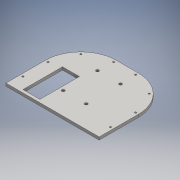
# Autodesk Inventor part: back_platform
Saved by Autodesk Inventor 2016 (Build 200138000, 138)
## iProperties
Created: 2015-09-09
Part Number: back_platform
Material: Generic
Document SubType Name: Modeling
Designer: oscar
Density: 1 g/cm^3
Appearance: Default
Author: oscar
Autodesk Inventor part; units mm, degrees
ref_plane "YZ Plane" through (0, 0, 0) normal (1, 0, 0) x (0, 1, 0)
ref_plane "XZ Plane" through (0, 0, 0) normal (0, 1, 0) x (-1, 0, 0)
ref_plane "XY Plane" through (0, 0, 0) normal (0, 0, 1) x (1, 0, 0)
sketch "Sketch1" plane through (0, 0, 0) normal (0, 0, 1) x (1, 0, 0)
  arc A0 (2041.1632, 1770.0189) -> (1915.1632, 1644.0189) centre (2041.1632, 1644.0189) ccw
  arc A1 (2245.1632, 1644.0189) -> (2119.1632, 1770.0189) centre (2119.1632, 1644.0189) ccw
  line L0 (1965.1632, 1655.0189) -> (1965.1632, 1515.0189)
  line L1 (2025.1632, 1655.0189) -> (2025.1632, 1515.0189)
  line L2 (1915.1632, 1505.0189) -> (2245.1632, 1505.0189)
  circle A2 centre (2041.1632, 1760.0189) radius 3
  circle A3 centre (2119.1632, 1760.0189) radius 3
  circle A4 centre (1925.1632, 1555.0189) radius 3
  line L3 (1960.1632, 1660.0189) -> (1960.1632, 1510.0189)
  line L4 (1960.1632, 1660.0189) -> (2030.1632, 1660.0189)
  line L5 (2030.1632, 1660.0189) -> (2030.1632, 1510.0189)
  circle A5 centre (2235.1632, 1555.0189) radius 3
  circle A6 centre (1925.1632, 1644.0189) radius 3
  circle A7 centre (2235.1632, 1644.0189) radius 3
  circle A8 centre (2039.352, 1704.8301) radius 5
  circle A9 centre (2120.9743, 1704.8301) radius 5
  circle A10 centre (2039.352, 1583.2077) radius 5
  circle A11 centre (2120.9743, 1583.2077) radius 5
  line L6 (1960.1632, 1510.0189) -> (2030.1632, 1510.0189)
  circle A12 centre (2201.1876, 1726.0433) radius 3
  circle A13 centre (1959.1388, 1726.0433) radius 3
  line L7 (2041.1632, 1770.0189) -> (2119.1632, 1770.0189)
  line L8 (2245.1632, 1644.0189) -> (2245.1632, 1505.0189)
  line L9 (1915.1632, 1644.0189) -> (1915.1632, 1505.0189)
  line L10 (1965.1632, 1655.0189) -> (2025.1632, 1655.0189)
  line L11 (1965.1632, 1515.0189) -> (2025.1632, 1515.0189)
  point P0 (0, 0)
  constraints: 24 end point, 14 centre point, 4 point on circle, 2 parallel, 2 perpendicular, 1 horizontal
extrude "Extrusion1" add sketch "Sketch1" along normal blind 10 contours L7 A1 L8 L2 L9 A0 | L4 L5 L6 L3
body "Solid1"
